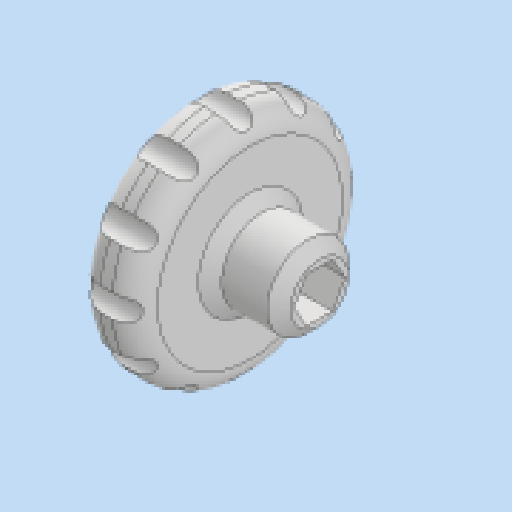
# Autodesk Inventor part: scroll_wheel
Saved by Autodesk Inventor 2024 (Build 280153000, 153)
## iProperties
Created: 2025-05-08
Part Number: scroll_wheel
Material: Generic
Document SubType Name: Modeling
Designer: XxPan
Density: 1 g/cm^3
Appearance: Default
Sheet Metal Rule: Default
Author: XxPan
Autodesk Inventor part; units mm, degrees
ref_plane "YZ Plane" through (0, 0, 0) normal (1, 0, 0) x (0, 1, 0)
ref_plane "XZ Plane" through (0, 0, 0) normal (0, 1, 0) x (-1, 0, 0)
ref_plane "XY Plane" through (0, 0, 0) normal (0, 0, 1) x (1, 0, 0)
sketch "Sketch1" plane through (0, 0, 0) normal (1, 0, 0) x (0, 1, 0)
  circle A0 centre (0, 0) radius 10
  dimension "d0" = 20
  constraints: 1 centre point, 1 coincident
  measures "d0" diameter of A0
extrude "Extrusion1" add sketch "Sketch1" along normal mid plane 5
sketch "Sketch2" plane through (2.5, 0, 0) normal (1, 0, 0) x (0, 0, -1)
  circle A0 centre (0, 0) radius 3.5
  dimension "d3" = 7
  constraints: 1 centre point, 1 coincident
  measures "d3" diameter of A0
extrude "Extrusion2" add sketch "Sketch2" along normal blind 6
sketch "Sketch3" plane through (-2.5, 0, 0) normal (-1, 0, 0) x (0, 0, 1)
  circle A0 centre (0, 0) radius 3.5 projected
  line L0 (1.1258, 1.95) -> (2.2517, 0)
  line L1 (2.2517, 0) -> (1.1258, -1.95)
  line L2 (1.1258, -1.95) -> (-1.1258, -1.95)
  line L3 (-1.1258, -1.95) -> (-2.2517, 0)
  line L4 (-2.2517, 0) -> (-1.1258, 1.95)
  line L5 (-1.1258, 1.95) -> (1.1258, 1.95)
  dimension "d6" = 3.9
  constraints: 12 end point, 1 coincident, 13 other
  measures "d6" distance between parallel lines of L2 L5
extrude "Extrusion3" cut sketch "Sketch3" against normal through all contours L0 L1 L2 L3 L4 L5
chamfer "Chamfer1" distance 1 angle 45 1 edges at (2.5, 0, 3.5)
fillet "Fillet1" radius 2 2 edges at (2.5, -10, 0) (-2.5, -10, 0)
chamfer "Chamfer2" distance 1 angle 45 6 edges at (-2.5, 0.975, -1.6887) (-2.5, 1.95, 0) (-2.5, 0.975, 1.6887) (-2.5, -0.975, 1.6887) (-2.5, -1.95, 0) (-2.5, -0.975, -1.6887)
sketch "Sketch5" plane through (0, 0, 0) normal (1, 0, 0) x (0, 1, 0)
  circle A0 centre (0, 0) radius 10 construction
  circle A1 centre (10, 0.0004) radius 1
  circle A2 centre (8.66, 5.0004) radius 1
  circle A3 centre (4.9996, 8.6605) radius 1
  circle A4 centre (-0.0004, 10) radius 1
  circle A5 centre (-5.0004, 8.66) radius 1
  circle A6 centre (-8.6605, 4.9996) radius 1
  circle A7 centre (-10, -0.0004) radius 1
  circle A8 centre (-8.66, -5.0004) radius 1
  circle A9 centre (-4.9996, -8.6605) radius 1
  circle A10 centre (0.0004, -10) radius 1
  circle A11 centre (5.0004, -8.66) radius 1
  circle A12 centre (8.6605, -4.9996) radius 1
  dimension "d27" = 2
  dimension "d30" = 360
  constraints: 12 centre point, 27 other
  measures "d27" diameter of A1
extrude "Extrusion4" cut sketch "Sketch5" along normal through all both and the other way through all
chamfer "Chamfer3" distance 1 angle 45 1 edges at (8.5, 0, 3.5)
equation "\"BendRadius\" = Thickness"
equation "\"BendReliefWidth\" = Thickness"
equation "\"BendReliefDepth\" = 0.5 * Thickness"
equation "\"CornerReliefSize\" = 4 * Thickness"
equation "\"MinimumRemnant\" = 2 * Thickness"
equation "\"TransitionRadius\" = BendRadius"
equation "\"JacobiRadiusSize\" = BendRadius"
equation "\"GapSize\" = Thickness"
equation "\"Thickness\" = 3.048"
body "Solid1"
